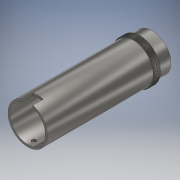
# Autodesk Inventor part: Body Tube
Saved by Autodesk Inventor 2018 (Build 220112000, 112)
## iProperties
Created: 2018-05-13
Part Number: Body Tube
Material: Steel, Mild
Document SubType Name: Modeling
Designer: Michel Gordillo
Density: 7.85 g/cm^3
Appearance: Semi-Polished
Author: Michel Gordillo
Autodesk Inventor part; units mm, degrees
ref_plane "YZ Plane" through (0, 0, 0) normal (1, 0, 0) x (0, 1, 0)
sketch "Sketch1" plane through (0, 0, 0) normal (0, 1, 0) x (-1, 0, 0)
  circle A0 centre (0, 0) radius 9.5
  circle A1 centre (0, 0) radius 8.5
  dimension "d0" = 19
  dimension "d1" = 17
  constraints: 2 centre point, 2 coincident
  measures "d0" diameter of A0
  measures "d1" diameter of A1
extrude "Extrusion1" add sketch "Sketch1" along normal blind 60
sketch "Sketch2" plane through (0, 60, 0) normal (0, 1, 0) x (1, 0, 0)
  circle A0 centre (0, 0) radius 9
  circle A1 centre (0, 0) radius 9.5
  dimension "d4" = 18
  constraints: 2 centre point, 2 coincident
  measures "d4" diameter of A0
extrude "Extrusion2" cut sketch "Sketch2" against normal blind 6
sketch "Sketch3" plane through (0, 54, 0) normal (0, 1, 0) x (1, 0, 0)
  circle A0 centre (0, 0) radius 10
  circle A1 centre (0, 0) radius 9.5
  line L0 (0, 0) -> (11.2327, 0) construction
  dimension "d7" = 20
  constraints: 2 centre point, 2 coincident, 2 end point, 1 horizontal
  measures "d7" diameter of A0
extrude "Extrusion3" add sketch "Sketch3" against normal blind 3
sketch "Sketch4" plane through (0, 54, 0) normal (0, 1, 0) x (1, 0, 0)
  line L0 (0, 0) -> (11.5066, -0.2511)
  line L1 (0, 0) -> (11.5093, 0) construction
  circle A0 centre (0, 0) radius 10 projected
  line L2 (9.9976, -0.2181) -> (9.8146, -0.1071)
  line L3 (9.8146, -0.1071) -> (10, 0)
  arc A1 (9.9976, -0.2181) -> (10, 0) centre (0, 0) ccw
  dimension "d16" = 1.25
  dimension "d19" = 30
  dimension "d21" = 30
  constraints: 8 end point, 4 point on circle, 2 point on line, 1 centre point, 1 coincident, 1 equal length, 1 horizontal
  measures "d16" angle of L0 L1
  measures "d19" angle of L1 L3
  measures "d21" angle of L0 L2
extrude "Extrusion4" cut sketch "Sketch4" against normal blind 3 contours A0 L2 L3 picked at (9.937, -0.1569)
pattern_circular "Circular Pattern1" count 288 over 360 about axis through (0, 54, 0) along (0, -1, 0) of "Extrusion4"
ref_plane "Work Plane2" through (0, 0, -8.5) normal (0, 0, -1) x (-1, 0, 0)
sketch "Sketch6" plane through (0, 0, -8.5) normal (0, 0, -1) x (-1, 0, 0)
  line L0 (-2, 51) -> (2, 51)
  line L1 (2, 51) -> (2, 30)
  line L2 (1, 29) -> (-1, 29)
  line L3 (-2, 30) -> (-2, 51)
  arc A0 (-2, 30) -> (-1, 29) centre (-1, 30) ccw
  arc A1 (1, 29) -> (2, 30) centre (1, 30) ccw
  point P0 (0, 0)
  point P1 (2, 29)
  point P2 (-2, 29)
  dimension "d27" = 4
  dimension "d28" = 22
  dimension "d29" = 1
  constraints: 8 end point, 4 point on circle, 4 point on line, 4 tangent, 2 centre point, 2 parallel, 1 equal radius, 1 horizontal, 1 perpendicular
  measures "d27" distance of point (2, 29) point (-2, 29)
  measures "d28" distance of L0.end point (2, 29)
  measures "d29" radius of A0
extrude "Extrusion5" add sketch "Sketch6" along normal blind 3
sketch "Sketch7" plane through (-2, 30, -9.2871) normal (-1, 0, 0) x (0, 0, 1)
  line L0 (-2.2129, 0) -> (-2.2129, 21) projected
  line L1 (-0.5, 21) -> (-2.2129, 21)
  line L2 (-2.2129, 21) -> (-2.2129, 11)
  line L3 (-2.2129, 11) -> (-0.5, 11)
  line L4 (-0.5, 11) -> (-0.5, 21)
  point P0 (9.2871, -30)
  dimension "d32" = 10
  constraints: 8 end point, 2 parallel, 1 horizontal, 1 perpendicular, 1 point on line
  measures "d32" distance of L2.end L1.end
extrude "Extrusion6" cut sketch "Sketch7" against normal up to next
sketch "Sketch8" plane through (-2, 30, -9.2871) normal (-1, 0, 0) x (0, 0, 1)
  line L0 (-2.2129, 11) -> (-2.2129, 0) projected
  line L1 (-2.2129, 11) -> (-2.2129, 10)
  line L2 (-2.2129, 10) -> (-1.3469, 10.5)
  line L3 (-2.188, 11) -> (-1.127, 11) construction
  line L4 (-2.2129, 11) -> (-0.5, 11) projected
  line L5 (-2.2129, 11) -> (-1.3469, 10.5)
  line L6 (-2.2129, 10) -> (-2.2129, 9)
  line L7 (-2.2129, 9) -> (-1.3469, 9.5)
  line L8 (-2.2129, 10) -> (-1.3469, 9.5)
  line L9 (-2.2129, 9) -> (-2.2129, 8)
  line L10 (-2.2129, 8) -> (-1.3469, 8.5)
  line L11 (-2.2129, 9) -> (-1.3469, 8.5)
  line L12 (-2.2129, 8) -> (-2.2129, 7)
  line L13 (-2.2129, 7) -> (-1.3469, 7.5)
  line L14 (-2.2129, 8) -> (-1.3469, 7.5)
  line L15 (-2.2129, 7) -> (-2.2129, 6)
  line L16 (-2.2129, 6) -> (-1.3469, 6.5)
  line L17 (-2.2129, 7) -> (-1.3469, 6.5)
  line L18 (-2.2129, 6) -> (-2.2129, 5)
  line L19 (-2.2129, 5) -> (-1.3469, 5.5)
  line L20 (-2.2129, 6) -> (-1.3469, 5.5)
  line L21 (-2.2129, 5) -> (-2.2129, 4)
  line L22 (-2.2129, 4) -> (-1.3469, 4.5)
  line L23 (-2.2129, 5) -> (-1.3469, 4.5)
  line L24 (-2.2129, 4) -> (-2.2129, 3)
  line L25 (-2.2129, 3) -> (-1.3469, 3.5)
  line L26 (-2.2129, 4) -> (-1.3469, 3.5)
  line L27 (-2.2129, 3) -> (-2.2129, 2)
  line L28 (-2.2129, 2) -> (-1.3469, 2.5)
  line L29 (-2.2129, 3) -> (-1.3469, 2.5)
  line L30 (-2.2129, 2) -> (-2.2129, 1)
  line L31 (-2.2129, 1) -> (-1.3469, 1.5)
  line L32 (-2.2129, 2) -> (-1.3469, 1.5)
  line L33 (-2.2129, 1) -> (-2.2129, 0)
  line L34 (-2.2129, 0) -> (-1.3469, 0.5)
  line L35 (-2.2129, 1) -> (-1.3469, 0.5)
  line L36 (-2.2129, 0) -> (-2.2129, -1)
  line L37 (-2.2129, -1) -> (-1.3469, -0.5)
  line L38 (-2.2129, 0) -> (-1.3469, -0.5)
  point P0 (9.2871, -30)
  point P1 (-2.188, 10)
  point P2 (-2.188, 9)
  point P3 (-2.188, 8)
  point P4 (-2.188, 7)
  point P5 (-2.188, 6)
  point P6 (-2.188, 5)
  point P7 (-2.188, 4)
  point P8 (-2.188, 3)
  point P9 (-2.188, 2)
  point P10 (-2.188, 1)
  point P11 (-2.188, 0)
  dimension "d35" = 1
  dimension "d36" = 60
  dimension "d38" = 60
  dimension "d41" = 1
  constraints: 74 end point, 1 horizontal, 1 point on line, 1 vertical, 77 other
  measures "d35" distance of L0.start L1.end
  measures "d36" angle of L2 L1
  measures "d38" angle of L5 L0
  measures "d41" distance of L0.start L6.start
extrude "Extrusion7" cut sketch "Sketch8" against normal up to next
ref_plane "Work Plane3" through (0, 0, 9.5) normal (0, 0, 1) x (1, 0, 0)
sketch "Sketch9" plane through (0, 0, 9.5) normal (0, 0, 1) x (1, 0, 0)
  line L0 (-9.5, 0) -> (9.5, 0) projected
  line L1 (-2.5, 0) -> (2.5, 0)
  line L2 (2.5, 0) -> (2.5, 5)
  line L3 (2.5, 5) -> (-2.5, 5)
  line L4 (-2.5, 5) -> (-2.5, 0)
  point P0 (0, 0)
  dimension "d48" = 5
  dimension "d49" = 5
  constraints: 8 end point, 2 parallel, 1 horizontal, 1 perpendicular, 1 point on line
  measures "d48" distance of L3.end L2.end
  measures "d49" distance of L2.end L1.end
extrude "Extrusion8" cut sketch "Sketch9" against normal up to next
sketch "Sketch10" plane through (0, 0, 9.5) normal (0, 0, 1) x (1, 0, 0)
  circle A0 centre (0, 3) radius 1
  point P0 (0, 0)
  dimension "d52" = 2
  constraints: 1 centre point
  measures "d52" diameter of A0
extrude "Extrusion9" cut sketch "Sketch10" against normal up to next
body "Solid1"
